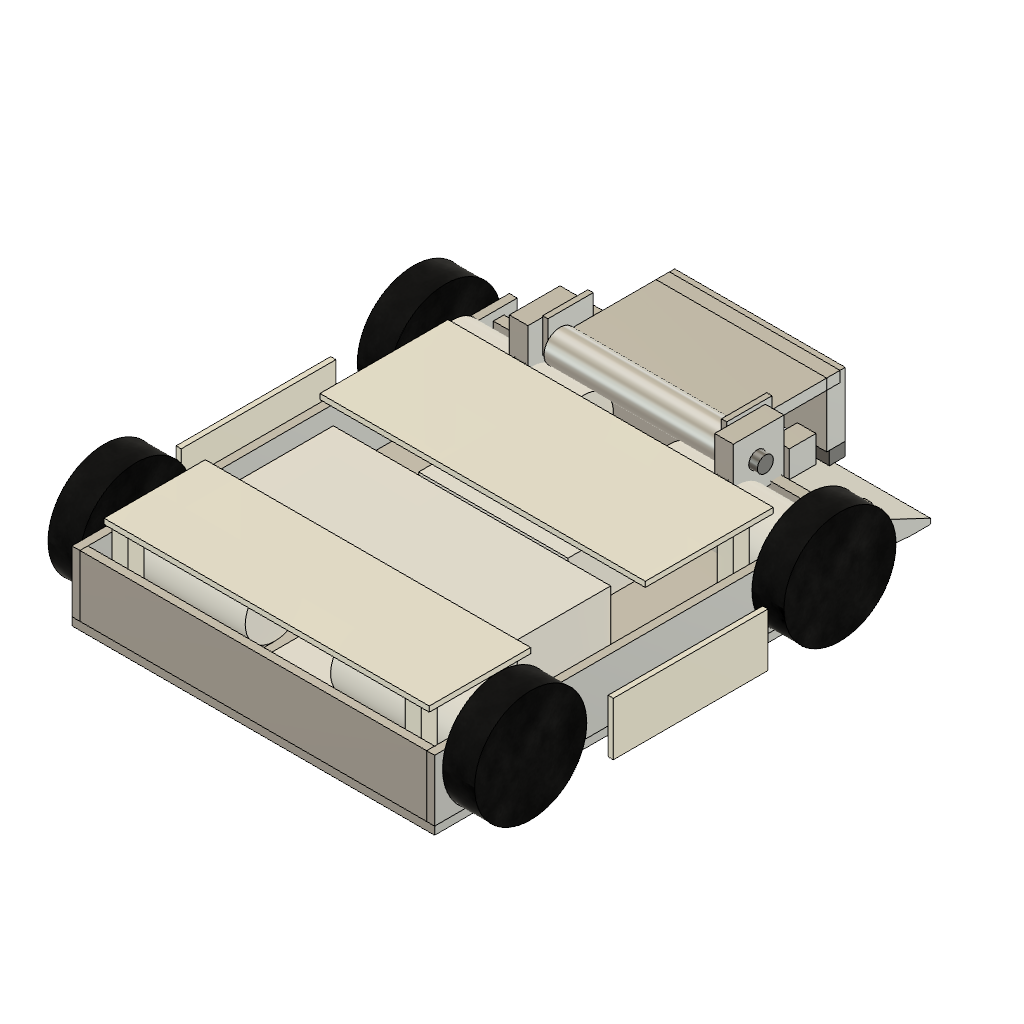
ROBOT_V3_Competition (Autodesk Fusion 360 design; units mm, degrees)
part number: 2026-09-24-19-02-37-994
part number: 2026-09-24-19-02-38-346
part number: 2026-09-24-19-02-38-350
part number: 2026-09-24-19-02-38-362
part number: 2026-09-24-19-02-38-371
part number: 2026-09-24-19-02-38-381
part number: 2026-09-24-19-02-38-392
part number: 2026-09-24-19-02-38-402
part number: 2026-09-24-19-02-38-411
part number: 2026-09-24-19-02-38-422
part number: 2026-09-24-19-02-38-425
part number: 2026-09-24-19-02-38-436
part number: 2026-09-24-19-02-38-447
part number: 2026-09-24-19-02-38-458
part number: 2026-09-24-19-02-38-470
part number: 2026-09-24-19-02-38-483
part number: 2026-09-24-19-02-38-496
part number: 2026-09-24-19-02-38-510
part number: 2026-09-24-19-02-38-525
part number: 2026-09-24-19-02-38-539
part number: 2026-09-24-19-02-38-554
part number: 2026-09-24-19-02-38-570
part number: 2026-09-24-19-02-38-586
part number: 2026-09-24-19-02-38-605
part number: 2026-09-24-19-02-38-624
part number: 2026-09-24-19-02-38-629
part number: 2026-09-24-19-02-38-655
part number: 2026-09-24-19-02-38-675
part number: 2026-09-24-19-02-38-696
part number: 2026-09-24-19-02-38-702
part number: 2026-09-24-19-02-38-753
part number: 2026-09-24-19-02-38-777
part number: 2026-09-24-19-02-38-800
part number: 2026-09-24-19-02-38-823
part number: 2026-09-24-19-02-38-847
part number: 2026-09-24-19-02-38-872
part number: 2026-09-24-19-02-38-933
part number: 2026-09-24-19-02-38-978
part number: 2026-09-24-19-02-39-006
part number: 2026-09-24-19-02-39-054
part number: 2026-09-24-19-02-39-085
part number: 2026-09-24-19-02-39-114
part number: 2026-09-24-19-02-39-145
part number: 2026-09-24-19-02-39-197
part number: 2026-09-24-19-02-39-235
part number: 2026-09-24-19-02-39-288
part number: 2026-09-24-19-02-39-435
part number: 2026-09-24-19-02-39-444
part number: 2026-09-24-19-02-39-476
part number: 2026-09-24-19-02-39-510
part number: 2026-09-24-19-02-39-543
part number: 2026-09-24-19-02-39-578
part number: 2026-09-24-19-02-39-612
part number: 2026-09-24-19-02-39-622
part number: 2026-09-24-19-02-39-658
part number: 2026-09-24-19-02-39-694
part number: 2026-09-24-19-02-39-731
part number: 2026-09-24-19-02-39-768
part number: 2026-09-24-19-02-39-806
Autodesk Fusion 360 part; units mm, degrees
sketch "Base_6061_3mm_Footprint" plane through (0, 0, 0) normal (0, 1, 0) x (1, 0, 0) in component "Base_6061_3mm"
  line L0 (-68, -82) -> (68, -82)
  line L1 (68, -82) -> (68, 82)
  line L2 (68, 82) -> (-68, 82)
  line L3 (-68, 82) -> (-68, -82)
extrude "Extrude1" add sketch "Base_6061_3mm_Footprint" along normal blind 3 from surface at 3 makes body 1 in component "Base_6061_3mm"
sketch "Side_Rail_L_6061_Footprint" plane through (0, 0, 0) normal (0, 1, 0) x (1, 0, 0) in component "Side_Rail_L_6061"
  line L0 (-68, -82) -> (-65, -82)
  line L1 (-65, -82) -> (-65, 82)
  line L2 (-65, 82) -> (-68, 82)
  line L3 (-68, 82) -> (-68, -82)
extrude "Extrude1'" add sketch "Side_Rail_L_6061_Footprint" along normal blind 23 from surface at 6 separate body makes body 2 in component "Side_Rail_L_6061"
sketch "Side_Rail_R_6061_Footprint" plane through (0, 0, 0) normal (0, 1, 0) x (1, 0, 0) in component "Side_Rail_R_6061"
  line L0 (65, -82) -> (68, -82)
  line L1 (68, -82) -> (68, 82)
  line L2 (68, 82) -> (65, 82)
  line L3 (65, 82) -> (65, -82)
extrude "Extrude1''" add sketch "Side_Rail_R_6061_Footprint" along normal blind 23 from surface at 6 separate body makes body 3 in component "Side_Rail_R_6061"
sketch "Rear_Cross_Member_6061_Footprint" plane through (0, 0, 0) normal (0, 1, 0) x (1, 0, 0) in component "Rear_Cross_Member_6061"
  line L0 (-65, -82) -> (65, -82)
  line L1 (65, -82) -> (65, -79)
  line L2 (65, -79) -> (-65, -79)
  line L3 (-65, -79) -> (-65, -82)
extrude "Extrude1'''" add sketch "Rear_Cross_Member_6061_Footprint" along normal blind 23 from surface at 6 separate body makes body 4 in component "Rear_Cross_Member_6061"
sketch "Front_Impact_Bulkhead_6061_Footprint" plane through (0, 0, 0) normal (0, 1, 0) x (1, 0, 0) in component "Front_Impact_Bulkhead_6061"
  line L0 (-62, 70) -> (62, 70)
  line L1 (62, 70) -> (62, 74)
  line L2 (62, 74) -> (-62, 74)
  line L3 (-62, 74) -> (-62, 70)
extrude "Extrude1''''" add sketch "Front_Impact_Bulkhead_6061_Footprint" along normal blind 23 from surface at 6 separate body makes body 5 in component "Front_Impact_Bulkhead_6061"
sketch "Front_Shear_Key_L_Footprint" plane through (0, 0, 0) normal (0, 1, 0) x (1, 0, 0) in component "Front_Shear_Key_L"
  line L0 (-60, 62) -> (-48, 62)
  line L1 (-48, 62) -> (-48, 70)
  line L2 (-48, 70) -> (-60, 70)
  line L3 (-60, 70) -> (-60, 62)
extrude "Extrude1'''''" add sketch "Front_Shear_Key_L_Footprint" along normal blind 18 from surface at 6 separate body makes body 6 in component "Front_Shear_Key_L"
sketch "Front_Shear_Key_R_Footprint" plane through (0, 0, 0) normal (0, 1, 0) x (1, 0, 0) in component "Front_Shear_Key_R"
  line L0 (48, 62) -> (60, 62)
  line L1 (60, 62) -> (60, 70)
  line L2 (60, 70) -> (48, 70)
  line L3 (48, 70) -> (48, 62)
extrude "Extrude1''''''" add sketch "Front_Shear_Key_R_Footprint" along normal blind 18 from surface at 6 separate body makes body 7 in component "Front_Shear_Key_R"
sketch "BBB_22mm_Gearmotor_ENVELOPE_L_Rear_Section" plane through (0, 0, 0) normal (1, 0, 0) x (0, 0, -1) in component "BBB_22mm_Gearmotor_ENVELOPE_L_Rear"
  circle A0 centre (-58, 23) radius 11
extrude "Extrude1'''''''" add sketch "BBB_22mm_Gearmotor_ENVELOPE_L_Rear_Section" along normal blind 49 from surface at -65 separate body makes body 8 in component "BBB_22mm_Gearmotor_ENVELOPE_L_Rear"
sketch "Wheel_42mm_ENVELOPE_L_Rear_Section" plane through (0, 0, 0) normal (1, 0, 0) x (0, 0, -1) in component "Wheel_42mm_ENVELOPE_L_Rear"
  circle A0 centre (-58, 23) radius 21
extrude "Extrude1''''''''" add sketch "Wheel_42mm_ENVELOPE_L_Rear_Section" along normal blind 12 from surface at -80 separate body makes body 9 in component "Wheel_42mm_ENVELOPE_L_Rear"
sketch "Axle_4mm_ENVELOPE_L_Rear_Section" plane through (0, 0, 0) normal (1, 0, 0) x (0, 0, -1) in component "Axle_4mm_ENVELOPE_L_Rear"
  circle A0 centre (-58, 23) radius 2
extrude "Extrude1'''''''''" add sketch "Axle_4mm_ENVELOPE_L_Rear_Section" along normal blind 9 from surface at -71 separate body makes body 10 in component "Axle_4mm_ENVELOPE_L_Rear"
sketch "BBB_22mm_Gearmotor_ENVELOPE_L_Front_Section" plane through (0, 0, 0) normal (1, 0, 0) x (0, 0, -1) in component "BBB_22mm_Gearmotor_ENVELOPE_L_Front"
  circle A0 centre (58, 23) radius 11
extrude "Extrude1''''''''''" add sketch "BBB_22mm_Gearmotor_ENVELOPE_L_Front_Section" along normal blind 49 from surface at -65 separate body makes body 11 in component "BBB_22mm_Gearmotor_ENVELOPE_L_Front"
sketch "Wheel_42mm_ENVELOPE_L_Front_Section" plane through (0, 0, 0) normal (1, 0, 0) x (0, 0, -1) in component "Wheel_42mm_ENVELOPE_L_Front"
  circle A0 centre (58, 23) radius 21
extrude "Extrude1'''''''''''" add sketch "Wheel_42mm_ENVELOPE_L_Front_Section" along normal blind 12 from surface at -80 separate body makes body 12 in component "Wheel_42mm_ENVELOPE_L_Front"
sketch "Axle_4mm_ENVELOPE_L_Front_Section" plane through (0, 0, 0) normal (1, 0, 0) x (0, 0, -1) in component "Axle_4mm_ENVELOPE_L_Front"
  circle A0 centre (58, 23) radius 2
extrude "Extrude1''''''''''''" add sketch "Axle_4mm_ENVELOPE_L_Front_Section" along normal blind 9 from surface at -71 separate body makes body 13 in component "Axle_4mm_ENVELOPE_L_Front"
sketch "BBB_22mm_Gearmotor_ENVELOPE_R_Rear_Section" plane through (0, 0, 0) normal (1, 0, 0) x (0, 0, -1) in component "BBB_22mm_Gearmotor_ENVELOPE_R_Rear"
  circle A0 centre (-58, 23) radius 11
extrude "Extrude1'''''''''''''" add sketch "BBB_22mm_Gearmotor_ENVELOPE_R_Rear_Section" along normal blind 49 from surface at 16 separate body makes body 14 in component "BBB_22mm_Gearmotor_ENVELOPE_R_Rear"
sketch "Wheel_42mm_ENVELOPE_R_Rear_Section" plane through (0, 0, 0) normal (1, 0, 0) x (0, 0, -1) in component "Wheel_42mm_ENVELOPE_R_Rear"
  circle A0 centre (-58, 23) radius 21
extrude "Extrude1''''''''''''''" add sketch "Wheel_42mm_ENVELOPE_R_Rear_Section" along normal blind 12 from surface at 68 separate body makes body 15 in component "Wheel_42mm_ENVELOPE_R_Rear"
sketch "Axle_4mm_ENVELOPE_R_Rear_Section" plane through (0, 0, 0) normal (1, 0, 0) x (0, 0, -1) in component "Axle_4mm_ENVELOPE_R_Rear"
  circle A0 centre (-58, 23) radius 2
extrude "Extrude1'''''''''''''''" add sketch "Axle_4mm_ENVELOPE_R_Rear_Section" along normal blind 9 from surface at 62 separate body makes body 16 in component "Axle_4mm_ENVELOPE_R_Rear"
sketch "BBB_22mm_Gearmotor_ENVELOPE_R_Front_Section" plane through (0, 0, 0) normal (1, 0, 0) x (0, 0, -1) in component "BBB_22mm_Gearmotor_ENVELOPE_R_Front"
  circle A0 centre (58, 23) radius 11
extrude "Extrude1''''''''''''''''" add sketch "BBB_22mm_Gearmotor_ENVELOPE_R_Front_Section" along normal blind 49 from surface at 16 separate body makes body 17 in component "BBB_22mm_Gearmotor_ENVELOPE_R_Front"
sketch "Wheel_42mm_ENVELOPE_R_Front_Section" plane through (0, 0, 0) normal (1, 0, 0) x (0, 0, -1) in component "Wheel_42mm_ENVELOPE_R_Front"
  circle A0 centre (58, 23) radius 21
extrude "Extrude1'''''''''''''''''" add sketch "Wheel_42mm_ENVELOPE_R_Front_Section" along normal blind 12 from surface at 68 separate body makes body 18 in component "Wheel_42mm_ENVELOPE_R_Front"
sketch "Axle_4mm_ENVELOPE_R_Front_Section" plane through (0, 0, 0) normal (1, 0, 0) x (0, 0, -1) in component "Axle_4mm_ENVELOPE_R_Front"
  circle A0 centre (58, 23) radius 2
extrude "Extrude1''''''''''''''''''" add sketch "Axle_4mm_ENVELOPE_R_Front_Section" along normal blind 9 from surface at 62 separate body makes body 19 in component "Axle_4mm_ENVELOPE_R_Front"
sketch "Replaceable_Side_Guard_L_Footprint" plane through (0, 0, 0) normal (0, 1, 0) x (1, 0, 0) in component "Replaceable_Side_Guard_L"
  line L0 (-82, -29) -> (-80, -29)
  line L1 (-80, -29) -> (-80, 29)
  line L2 (-80, 29) -> (-82, 29)
  line L3 (-82, 29) -> (-82, -29)
extrude "Extrude1'''''''''''''''''''" add sketch "Replaceable_Side_Guard_L_Footprint" along normal blind 20 from surface at 8 separate body makes body 20 in component "Replaceable_Side_Guard_L"
sketch "Replaceable_Side_Guard_R_Footprint" plane through (0, 0, 0) normal (0, 1, 0) x (1, 0, 0) in component "Replaceable_Side_Guard_R"
  line L0 (80, -29) -> (82, -29)
  line L1 (82, -29) -> (82, 29)
  line L2 (82, 29) -> (80, 29)
  line L3 (80, 29) -> (80, -29)
extrude "Extrude1''''''''''''''''''''" add sketch "Replaceable_Side_Guard_R_Footprint" along normal blind 20 from surface at 8 separate body makes body 21 in component "Replaceable_Side_Guard_R"
sketch "Plow_Ramp_Profile" plane through (0, 0, 0) normal (1, 0, 0) x (0, 0, -1) in component "Bolt_On_Full_Width_Plow_6061"
  line L0 (74, 6) -> (74, 23)
  line L1 (74, 23) -> (112, 5)
  line L2 (112, 5) -> (112, 3)
  line L3 (112, 3) -> (104, 3)
  line L4 (104, 3) -> (74, 6)
extrude "Extrude1'''''''''''''''''''''" add sketch "Plow_Ramp_Profile" along normal blind 120 from surface at -60 separate body makes body 22 in component "Bolt_On_Full_Width_Plow_6061"
sketch "Plow_Bolt_Land_L_Footprint" plane through (0, 0, 0) normal (0, 1, 0) x (1, 0, 0) in component "Plow_Bolt_Land_L"
  line L0 (-54, 65) -> (-44, 65)
  line L1 (-44, 65) -> (-44, 74)
  line L2 (-44, 74) -> (-54, 74)
  line L3 (-54, 74) -> (-54, 65)
extrude "Extrude1''''''''''''''''''''''" add sketch "Plow_Bolt_Land_L_Footprint" along normal blind 16 from surface at 6 separate body makes body 23 in component "Plow_Bolt_Land_L"
sketch "Plow_Bolt_Land_R_Footprint" plane through (0, 0, 0) normal (0, 1, 0) x (1, 0, 0) in component "Plow_Bolt_Land_R"
  line L0 (44, 65) -> (54, 65)
  line L1 (54, 65) -> (54, 74)
  line L2 (54, 74) -> (44, 74)
  line L3 (44, 74) -> (44, 65)
extrude "Extrude1'''''''''''''''''''''''" add sketch "Plow_Bolt_Land_R_Footprint" along normal blind 16 from surface at 6 separate body makes body 24 in component "Plow_Bolt_Land_R"
sketch "Clamp_Jaw_Plate_6061_Footprint" plane through (0, 0, 0) normal (0, 1, 0) x (1, 0, 0) in component "Clamp_Jaw_Plate_6061"
  line L0 (-32, 65) -> (32, 65)
  line L1 (32, 65) -> (32, 106)
  line L2 (32, 106) -> (-32, 106)
  line L3 (-32, 106) -> (-32, 65)
extrude "Extrude1''''''''''''''''''''''''" add sketch "Clamp_Jaw_Plate_6061_Footprint" along normal blind 4 from surface at 38 separate body makes body 25 in component "Clamp_Jaw_Plate_6061"
sketch "Hinge_Boss_Section" plane through (0, 0, 0) normal (1, 0, 0) x (0, 0, -1) in component "Clamp_Jaw_Plate_6061"
  circle A0 centre (65, 38.5) radius 6
extrude "Extrude2" add sketch "Hinge_Boss_Section" along normal blind 64 from surface at -32 bodies 25 in component "Clamp_Jaw_Plate_6061"
sketch "Hinge_Bore_6p4mm" plane through (0, 0, 0) normal (1, 0, 0) x (0, 0, -1) in component "Clamp_Jaw_Plate_6061"
  circle A0 centre (65, 38.5) radius 3.2
extrude "Extrude3" cut sketch "Hinge_Bore_6p4mm" along normal mid plane 200 bodies 25 in component "Clamp_Jaw_Plate_6061"
sketch "Clamp_Downturned_Tip_6061_Footprint" plane through (0, 0, 0) normal (0, 1, 0) x (1, 0, 0) in component "Clamp_Downturned_Tip_6061"
  line L0 (-32, 101) -> (32, 101)
  line L1 (32, 101) -> (32, 108)
  line L2 (32, 108) -> (-32, 108)
  line L3 (-32, 108) -> (-32, 101)
extrude "Extrude1'''''''''''''''''''''''''" add sketch "Clamp_Downturned_Tip_6061_Footprint" along normal blind 24 from surface at 18 separate body makes body 26 in component "Clamp_Downturned_Tip_6061"
sketch "Replaceable_Clamp_Tooth_1_Steel_Footprint" plane through (0, 0, 0) normal (0, 1, 0) x (1, 0, 0) in component "Replaceable_Clamp_Tooth_1_Steel"
  line L0 (-28, 106) -> (-20, 106)
  line L1 (-20, 106) -> (-20, 112)
  line L2 (-20, 112) -> (-28, 112)
  line L3 (-28, 112) -> (-28, 106)
extrude "Extrude1''''''''''''''''''''''''''" add sketch "Replaceable_Clamp_Tooth_1_Steel_Footprint" along normal blind 11 from surface at 9 separate body makes body 27 in component "Replaceable_Clamp_Tooth_1_Steel"
sketch "Replaceable_Clamp_Tooth_2_Steel_Footprint" plane through (0, 0, 0) normal (0, 1, 0) x (1, 0, 0) in component "Replaceable_Clamp_Tooth_2_Steel"
  line L0 (-4, 106) -> (4, 106)
  line L1 (4, 106) -> (4, 112)
  line L2 (4, 112) -> (-4, 112)
  line L3 (-4, 112) -> (-4, 106)
extrude "Extrude1'''''''''''''''''''''''''''" add sketch "Replaceable_Clamp_Tooth_2_Steel_Footprint" along normal blind 11 from surface at 9 separate body makes body 28 in component "Replaceable_Clamp_Tooth_2_Steel"
sketch "Replaceable_Clamp_Tooth_3_Steel_Footprint" plane through (0, 0, 0) normal (0, 1, 0) x (1, 0, 0) in component "Replaceable_Clamp_Tooth_3_Steel"
  line L0 (20, 106) -> (28, 106)
  line L1 (28, 106) -> (28, 112)
  line L2 (28, 112) -> (20, 112)
  line L3 (20, 112) -> (20, 106)
extrude "Extrude1''''''''''''''''''''''''''''" add sketch "Replaceable_Clamp_Tooth_3_Steel_Footprint" along normal blind 11 from surface at 9 separate body makes body 29 in component "Replaceable_Clamp_Tooth_3_Steel"
sketch "Clamp_Torque_Arm_L_Footprint" plane through (0, 0, 0) normal (0, 1, 0) x (1, 0, 0) in component "Clamp_Torque_Arm_L"
  line L0 (-34.5, 61) -> (-32.5, 61)
  line L1 (-32.5, 61) -> (-32.5, 78)
  line L2 (-32.5, 78) -> (-34.5, 78)
  line L3 (-34.5, 78) -> (-34.5, 61)
extrude "Extrude1'''''''''''''''''''''''''''''" add sketch "Clamp_Torque_Arm_L_Footprint" along normal blind 13 from surface at 36 separate body makes body 30 in component "Clamp_Torque_Arm_L"
sketch "Clamp_Torque_Arm_R_Footprint" plane through (0, 0, 0) normal (0, 1, 0) x (1, 0, 0) in component "Clamp_Torque_Arm_R"
  line L0 (32.5, 61) -> (34.5, 61)
  line L1 (34.5, 61) -> (34.5, 78)
  line L2 (34.5, 78) -> (32.5, 78)
  line L3 (32.5, 78) -> (32.5, 61)
extrude "Extrude1''''''''''''''''''''''''''''''" add sketch "Clamp_Torque_Arm_R_Footprint" along normal blind 13 from surface at 36 separate body makes body 31 in component "Clamp_Torque_Arm_R"
sketch "Torque_Arm_Pin_Bore_L" plane through (0, 0, 0) normal (1, 0, 0) x (0, 0, -1) in component "Clamp_Torque_Arm_L"
  circle A0 centre (65, 38.5) radius 3.2
extrude "Extrude2'" cut sketch "Torque_Arm_Pin_Bore_L" along normal mid plane 200 bodies 30 in component "Clamp_Torque_Arm_L"
sketch "Torque_Arm_Pin_Bore_R" plane through (0, 0, 0) normal (1, 0, 0) x (0, 0, -1) in component "Clamp_Torque_Arm_R"
  circle A0 centre (65, 38.5) radius 3.2
extrude "Extrude2''" cut sketch "Torque_Arm_Pin_Bore_R" along normal mid plane 200 bodies 31 in component "Clamp_Torque_Arm_R"
sketch "Hinge_Cheek_L_Footprint" plane through (0, 0, 0) normal (0, 1, 0) x (1, 0, 0) in component "Hinge_Cheek_L"
  line L0 (-42, 56) -> (-35, 56)
  line L1 (-35, 56) -> (-35, 75)
  line L2 (-35, 75) -> (-42, 75)
  line L3 (-42, 75) -> (-42, 56)
extrude "Extrude1'''''''''''''''''''''''''''''''" add sketch "Hinge_Cheek_L_Footprint" along normal blind 20 from surface at 28 separate body makes body 32 in component "Hinge_Cheek_L"
sketch "Pin_Bore_6p4mm" plane through (0, 0, 0) normal (1, 0, 0) x (0, 0, -1) in component "Hinge_Cheek_L"
  circle A0 centre (65, 38.5) radius 3.2
extrude "Extrude2'''" cut sketch "Pin_Bore_6p4mm" along normal mid plane 200 bodies 32 in component "Hinge_Cheek_L"
sketch "Downward_Hard_Stop_L_Footprint" plane through (0, 0, 0) normal (0, 1, 0) x (1, 0, 0) in component "Downward_Hard_Stop_L"
  line L0 (-42, 77) -> (-35, 77)
  line L1 (-35, 77) -> (-35, 87)
  line L2 (-35, 87) -> (-42, 87)
  line L3 (-42, 87) -> (-42, 77)
extrude "Extrude1''''''''''''''''''''''''''''''''" add sketch "Downward_Hard_Stop_L_Footprint" along normal blind 10 from surface at 26 separate body makes body 33 in component "Downward_Hard_Stop_L"
sketch "Hinge_Cheek_R_Footprint" plane through (0, 0, 0) normal (0, 1, 0) x (1, 0, 0) in component "Hinge_Cheek_R"
  line L0 (35, 56) -> (42, 56)
  line L1 (42, 56) -> (42, 75)
  line L2 (42, 75) -> (35, 75)
  line L3 (35, 75) -> (35, 56)
extrude "Extrude1'''''''''''''''''''''''''''''''''" add sketch "Hinge_Cheek_R_Footprint" along normal blind 20 from surface at 28 separate body makes body 34 in component "Hinge_Cheek_R"
sketch "Pin_Bore_6p4mm (2)" plane through (0, 0, 0) normal (1, 0, 0) x (0, 0, -1) in component "Hinge_Cheek_R"
  circle A0 centre (65, 38.5) radius 3.2
extrude "Extrude2''''" cut sketch "Pin_Bore_6p4mm (2)" along normal mid plane 200 bodies 34 in component "Hinge_Cheek_R"
sketch "Downward_Hard_Stop_R_Footprint" plane through (0, 0, 0) normal (0, 1, 0) x (1, 0, 0) in component "Downward_Hard_Stop_R"
  line L0 (35, 77) -> (42, 77)
  line L1 (42, 77) -> (42, 87)
  line L2 (42, 87) -> (35, 87)
  line L3 (35, 87) -> (35, 77)
extrude "Extrude1''''''''''''''''''''''''''''''''''" add sketch "Downward_Hard_Stop_R_Footprint" along normal blind 10 from surface at 26 separate body makes body 35 in component "Downward_Hard_Stop_R"
sketch "Hinge_Pin_6mm_ENVELOPE_Section" plane through (0, 0, 0) normal (1, 0, 0) x (0, 0, -1) in component "Hinge_Pin_6mm_ENVELOPE"
  circle A0 centre (65, 38.5) radius 3
extrude "Extrude1'''''''''''''''''''''''''''''''''''" add sketch "Hinge_Pin_6mm_ENVELOPE_Section" along normal blind 90 from surface at -45 separate body makes body 36 in component "Hinge_Pin_6mm_ENVELOPE"
sketch "Repeat_40kg_Servo_ENVELOPE_Footprint" plane through (0, 0, 0) normal (0, 1, 0) x (1, 0, 0) in component "Repeat_40kg_Servo_ENVELOPE"
  line L0 (-28, 8) -> (28, 8)
  line L1 (28, 8) -> (28, 53)
  line L2 (28, 53) -> (-28, 53)
  line L3 (-28, 53) -> (-28, 8)
extrude "Extrude1''''''''''''''''''''''''''''''''''''" add sketch "Repeat_40kg_Servo_ENVELOPE_Footprint" along normal blind 20 from surface at 8 separate body makes body 37 in component "Repeat_40kg_Servo_ENVELOPE"
sketch "Servo_Output_Horn_6061_Section" plane through (0, 0, 0) normal (1, 0, 0) x (0, 0, -1) in component "Servo_Output_Horn_6061"
  circle A0 centre (51, 24) radius 6
extrude "Extrude1'''''''''''''''''''''''''''''''''''''" add sketch "Servo_Output_Horn_6061_Section" along normal blind 68 from surface at -34 separate body makes body 38 in component "Servo_Output_Horn_6061"
sketch "Servo_Output_Bore_3mm" plane through (0, 0, 0) normal (1, 0, 0) x (0, 0, -1) in component "Servo_Output_Horn_6061"
  circle A0 centre (51, 24) radius 1.5
extrude "Extrude2'''''" cut sketch "Servo_Output_Bore_3mm" along normal mid plane 200 bodies 38 in component "Servo_Output_Horn_6061"
sketch "Sketch1" plane through (0, 0, 0) normal (1, 0, 0) x (0, 0, -1) in component "Clamp_Linkage_L"
  line L0 (49.427, 29.9431) -> (70.427, 46.9431)
  line L1 (70.427, 46.9431) -> (73.573, 43.0569)
  line L2 (73.573, 43.0569) -> (52.573, 26.0569)
  line L3 (52.573, 26.0569) -> (49.427, 29.9431)
extrude "Extrude1''''''''''''''''''''''''''''''''''''''" add sketch "Sketch1" along normal blind 4 from surface at -40 separate body makes body 39 in component "Clamp_Linkage_L"
sketch "Sketch1 (2)" plane through (0, 0, 0) normal (1, 0, 0) x (0, 0, -1) in component "Clamp_Linkage_R"
  line L0 (49.427, 29.9431) -> (70.427, 46.9431)
  line L1 (70.427, 46.9431) -> (73.573, 43.0569)
  line L2 (73.573, 43.0569) -> (52.573, 26.0569)
  line L3 (52.573, 26.0569) -> (49.427, 29.9431)
extrude "Extrude1'''''''''''''''''''''''''''''''''''''''" add sketch "Sketch1 (2)" along normal blind 4 from surface at 36 separate body makes body 40 in component "Clamp_Linkage_R"
sketch "Servo_Linkage_Sweep_ENVELOPE_Footprint" plane through (0, 0, 0) normal (0, 1, 0) x (1, 0, 0) in component "Servo_Linkage_Sweep_ENVELOPE"
  line L0 (-9, 48) -> (9, 48)
  line L1 (9, 48) -> (9, 75)
  line L2 (9, 75) -> (-9, 75)
  line L3 (-9, 75) -> (-9, 48)
extrude "Extrude1''''''''''''''''''''''''''''''''''''''''" add sketch "Servo_Linkage_Sweep_ENVELOPE_Footprint" along normal blind 22 from surface at 28 separate body makes body 41 in component "Servo_Linkage_Sweep_ENVELOPE"
sketch "3S_Battery_104x35x27_ENVELOPE_Footprint" plane through (0, 0, 0) normal (0, 1, 0) x (1, 0, 0) in component "3S_Battery_104x35x27_ENVELOPE"
  line L0 (-52, -35) -> (52, -35)
  line L1 (52, -35) -> (52, 0)
  line L2 (52, 0) -> (-52, 0)
  line L3 (-52, 0) -> (-52, -35)
extrude "Extrude1'''''''''''''''''''''''''''''''''''''''''" add sketch "3S_Battery_104x35x27_ENVELOPE_Footprint" along normal blind 27 from surface at 8 separate body makes body 42 in component "3S_Battery_104x35x27_ENVELOPE"
sketch "Dual_ESC_ENVELOPE_Footprint" plane through (0, 0, 0) normal (0, 1, 0) x (1, 0, 0) in component "Dual_ESC_ENVELOPE"
  line L0 (-12, -72) -> (12, -72)
  line L1 (12, -72) -> (12, -52)
  line L2 (12, -52) -> (-12, -52)
  line L3 (-12, -52) -> (-12, -72)
extrude "Extrude1''''''''''''''''''''''''''''''''''''''''''" add sketch "Dual_ESC_ENVELOPE_Footprint" along normal blind 5 from surface at 8 separate body makes body 43 in component "Dual_ESC_ENVELOPE"
sketch "Receiver_ENVELOPE_Footprint" plane through (0, 0, 0) normal (0, 1, 0) x (1, 0, 0) in component "Receiver_ENVELOPE"
  line L0 (-48, -72) -> (-20, -72)
  line L1 (-20, -72) -> (-20, -54)
  line L2 (-20, -54) -> (-48, -54)
  line L3 (-48, -54) -> (-48, -72)
extrude "Extrude1'''''''''''''''''''''''''''''''''''''''''''" add sketch "Receiver_ENVELOPE_Footprint" along normal blind 6 from surface at 8 separate body makes body 44 in component "Receiver_ENVELOPE"
sketch "UBEC_ENVELOPE_Footprint" plane through (0, 0, 0) normal (0, 1, 0) x (1, 0, 0) in component "UBEC_ENVELOPE"
  line L0 (20, -72) -> (48, -72)
  line L1 (48, -72) -> (48, -54)
  line L2 (48, -54) -> (20, -54)
  line L3 (20, -54) -> (20, -72)
extrude "Extrude1''''''''''''''''''''''''''''''''''''''''''''" add sketch "UBEC_ENVELOPE_Footprint" along normal blind 7 from surface at 8 separate body makes body 45 in component "UBEC_ENVELOPE"
sketch "Power_Switch_ENVELOPE_Footprint" plane through (0, 0, 0) normal (0, 1, 0) x (1, 0, 0) in component "Power_Switch_ENVELOPE"
  line L0 (38, -65) -> (56, -65)
  line L1 (56, -65) -> (56, -45)
  line L2 (56, -45) -> (38, -45)
  line L3 (38, -45) -> (38, -65)
extrude "Extrude1'''''''''''''''''''''''''''''''''''''''''''''" add sketch "Power_Switch_ENVELOPE_Footprint" along normal blind 16 from surface at 9 separate body makes body 46 in component "Power_Switch_ENVELOPE"
sketch "Cover_Standoff_L_Rear_Footprint" plane through (0, 0, 0) normal (0, 1, 0) x (1, 0, 0) in component "Cover_Standoff_L_Rear"
  line L0 (-58, -77) -> (-52, -77)
  line L1 (-52, -77) -> (-52, -71)
  line L2 (-52, -71) -> (-58, -71)
  line L3 (-58, -71) -> (-58, -77)
extrude "Extrude1''''''''''''''''''''''''''''''''''''''''''''''" add sketch "Cover_Standoff_L_Rear_Footprint" along normal blind 31 from surface at 6 separate body makes body 47 in component "Cover_Standoff_L_Rear"
sketch "Cover_Standoff_L_Front_Footprint" plane through (0, 0, 0) normal (0, 1, 0) x (1, 0, 0) in component "Cover_Standoff_L_Front"
  line L0 (-58, 40) -> (-52, 40)
  line L1 (-52, 40) -> (-52, 46)
  line L2 (-52, 46) -> (-58, 46)
  line L3 (-58, 46) -> (-58, 40)
extrude "Extrude1'''''''''''''''''''''''''''''''''''''''''''''''" add sketch "Cover_Standoff_L_Front_Footprint" along normal blind 31 from surface at 6 separate body makes body 48 in component "Cover_Standoff_L_Front"
sketch "Cover_Standoff_R_Rear_Footprint" plane through (0, 0, 0) normal (0, 1, 0) x (1, 0, 0) in component "Cover_Standoff_R_Rear"
  line L0 (52, -77) -> (58, -77)
  line L1 (58, -77) -> (58, -71)
  line L2 (58, -71) -> (52, -71)
  line L3 (52, -71) -> (52, -77)
extrude "Extrude1''''''''''''''''''''''''''''''''''''''''''''''''" add sketch "Cover_Standoff_R_Rear_Footprint" along normal blind 31 from surface at 6 separate body makes body 49 in component "Cover_Standoff_R_Rear"
sketch "Cover_Standoff_R_Front_Footprint" plane through (0, 0, 0) normal (0, 1, 0) x (1, 0, 0) in component "Cover_Standoff_R_Front"
  line L0 (52, 40) -> (58, 40)
  line L1 (58, 40) -> (58, 46)
  line L2 (58, 46) -> (52, 46)
  line L3 (52, 46) -> (52, 40)
extrude "Extrude1'''''''''''''''''''''''''''''''''''''''''''''''''" add sketch "Cover_Standoff_R_Front_Footprint" along normal blind 31 from surface at 6 separate body makes body 50 in component "Cover_Standoff_R_Front"
sketch "Rear_Service_Lid_2mm_Footprint" plane through (0, 0, 0) normal (0, 1, 0) x (1, 0, 0) in component "Rear_Service_Lid_2mm"
  line L0 (-61, -77) -> (61, -77)
  line L1 (61, -77) -> (61, -39)
  line L2 (61, -39) -> (-61, -39)
  line L3 (-61, -39) -> (-61, -77)
extrude "Extrude1''''''''''''''''''''''''''''''''''''''''''''''''''" add sketch "Rear_Service_Lid_2mm_Footprint" along normal blind 2 from surface at 37 separate body makes body 51 in component "Rear_Service_Lid_2mm"
sketch "Center_Service_Lid_2mm_Footprint" plane through (0, 0, 0) normal (0, 1, 0) x (1, 0, 0) in component "Center_Service_Lid_2mm"
  line L0 (-61, 4) -> (61, 4)
  line L1 (61, 4) -> (61, 52)
  line L2 (61, 52) -> (-61, 52)
  line L3 (-61, 52) -> (-61, 4)
extrude "Extrude1'''''''''''''''''''''''''''''''''''''''''''''''''''" add sketch "Center_Service_Lid_2mm_Footprint" along normal blind 2 from surface at 37 separate body makes body 52 in component "Center_Service_Lid_2mm"
component "01_Low_Tub_Chassis" placed x (1, 0, 0) y (0, 1, 0) z (0, 0, 1) at (0, 0, 0)
component "02_Four_Wheel_Drive" placed x (1, 0, 0) y (0, 1, 0) z (0, 0, 1) at (0, 0, 0)
component "03_Front_Impact_Module" placed x (1, 0, 0) y (0, 1, 0) z (0, 0, 1) at (0, 0, 0)
component "04_Protected_Clamp_Weapon" placed x (1, 0, 0) y (0, 1, 0) z (0, 0, 1) at (0, 0, 0)
component "05_Protected_Electronics_ENVELOPES" placed x (1, 0, 0) y (0, 1, 0) z (0, 0, 1) at (0, 0, 0)
component "06_Removable_Covers" placed x (1, 0, 0) y (0, 1, 0) z (0, 0, 1) at (0, 0, 0)
component "Base_6061_3mm" placed x (1, 0, 0) y (0, 1, 0) z (0, 0, 1) at (0, 0, 0) in component "01_Low_Tub_Chassis"
component "Side_Rail_L_6061" placed x (1, 0, 0) y (0, 1, 0) z (0, 0, 1) at (0, 0, 0) in component "01_Low_Tub_Chassis"
component "Side_Rail_R_6061" placed x (1, 0, 0) y (0, 1, 0) z (0, 0, 1) at (0, 0, 0) in component "01_Low_Tub_Chassis"
component "Rear_Cross_Member_6061" placed x (1, 0, 0) y (0, 1, 0) z (0, 0, 1) at (0, 0, 0) in component "01_Low_Tub_Chassis"
component "Front_Impact_Bulkhead_6061" placed x (1, 0, 0) y (0, 1, 0) z (0, 0, 1) at (0, 0, 0) in component "01_Low_Tub_Chassis"
component "Front_Shear_Key_L" placed x (1, 0, 0) y (0, 1, 0) z (0, 0, 1) at (0, 0, 0) in component "01_Low_Tub_Chassis"
component "Front_Shear_Key_R" placed x (1, 0, 0) y (0, 1, 0) z (0, 0, 1) at (0, 0, 0) in component "01_Low_Tub_Chassis"
component "BBB_22mm_Gearmotor_ENVELOPE_L_Rear" placed x (1, 0, 0) y (0, 1, 0) z (0, 0, 1) at (0, 0, 0) in component "02_Four_Wheel_Drive"
component "Wheel_42mm_ENVELOPE_L_Rear" placed x (1, 0, 0) y (0, 1, 0) z (0, 0, 1) at (0, 0, 0) in component "02_Four_Wheel_Drive"
component "Axle_4mm_ENVELOPE_L_Rear" placed x (1, 0, 0) y (0, 1, 0) z (0, 0, 1) at (0, 0, 0) in component "02_Four_Wheel_Drive"
component "BBB_22mm_Gearmotor_ENVELOPE_L_Front" placed x (1, 0, 0) y (0, 1, 0) z (0, 0, 1) at (0, 0, 0) in component "02_Four_Wheel_Drive"
component "Wheel_42mm_ENVELOPE_L_Front" placed x (1, 0, 0) y (0, 1, 0) z (0, 0, 1) at (0, 0, 0) in component "02_Four_Wheel_Drive"
component "Axle_4mm_ENVELOPE_L_Front" placed x (1, 0, 0) y (0, 1, 0) z (0, 0, 1) at (0, 0, 0) in component "02_Four_Wheel_Drive"
component "BBB_22mm_Gearmotor_ENVELOPE_R_Rear" placed x (1, 0, 0) y (0, 1, 0) z (0, 0, 1) at (0, 0, 0) in component "02_Four_Wheel_Drive"
component "Wheel_42mm_ENVELOPE_R_Rear" placed x (1, 0, 0) y (0, 1, 0) z (0, 0, 1) at (0, 0, 0) in component "02_Four_Wheel_Drive"
component "Axle_4mm_ENVELOPE_R_Rear" placed x (1, 0, 0) y (0, 1, 0) z (0, 0, 1) at (0, 0, 0) in component "02_Four_Wheel_Drive"
component "BBB_22mm_Gearmotor_ENVELOPE_R_Front" placed x (1, 0, 0) y (0, 1, 0) z (0, 0, 1) at (0, 0, 0) in component "02_Four_Wheel_Drive"
component "Wheel_42mm_ENVELOPE_R_Front" placed x (1, 0, 0) y (0, 1, 0) z (0, 0, 1) at (0, 0, 0) in component "02_Four_Wheel_Drive"
component "Axle_4mm_ENVELOPE_R_Front" placed x (1, 0, 0) y (0, 1, 0) z (0, 0, 1) at (0, 0, 0) in component "02_Four_Wheel_Drive"
component "Replaceable_Side_Guard_L" placed x (1, 0, 0) y (0, 1, 0) z (0, 0, 1) at (0, 0, 0) in component "02_Four_Wheel_Drive"
component "Replaceable_Side_Guard_R" placed x (1, 0, 0) y (0, 1, 0) z (0, 0, 1) at (0, 0, 0) in component "02_Four_Wheel_Drive"
component "Bolt_On_Full_Width_Plow_6061" placed x (1, 0, 0) y (0, 1, 0) z (0, 0, 1) at (0, 0, 0) in component "03_Front_Impact_Module"
component "Plow_Bolt_Land_L" placed x (1, 0, 0) y (0, 1, 0) z (0, 0, 1) at (0, 0, 0) in component "03_Front_Impact_Module"
component "Plow_Bolt_Land_R" placed x (1, 0, 0) y (0, 1, 0) z (0, 0, 1) at (0, 0, 0) in component "03_Front_Impact_Module"
component "Clamp_Jaw_Plate_6061" placed x (1, 0, 0) y (0, 1, 0) z (0, 0, 1) at (0, 0, 0) in component "04_Protected_Clamp_Weapon"
component "Clamp_Downturned_Tip_6061" placed x (1, 0, 0) y (0, 1, 0) z (0, 0, 1) at (0, 0, 0) in component "04_Protected_Clamp_Weapon"
component "Replaceable_Clamp_Tooth_1_Steel" placed x (1, 0, 0) y (0, 1, 0) z (0, 0, 1) at (0, 0, 0) in component "04_Protected_Clamp_Weapon"
component "Replaceable_Clamp_Tooth_2_Steel" placed x (1, 0, 0) y (0, 1, 0) z (0, 0, 1) at (0, 0, 0) in component "04_Protected_Clamp_Weapon"
component "Replaceable_Clamp_Tooth_3_Steel" placed x (1, 0, 0) y (0, 1, 0) z (0, 0, 1) at (0, 0, 0) in component "04_Protected_Clamp_Weapon"
component "Clamp_Torque_Arm_L" placed x (1, 0, 0) y (0, 1, 0) z (0, 0, 1) at (0, 0, 0) in component "04_Protected_Clamp_Weapon"
component "Clamp_Torque_Arm_R" placed x (1, 0, 0) y (0, 1, 0) z (0, 0, 1) at (0, 0, 0) in component "04_Protected_Clamp_Weapon"
component "Hinge_Cheek_L" placed x (1, 0, 0) y (0, 1, 0) z (0, 0, 1) at (0, 0, 0) in component "04_Protected_Clamp_Weapon"
component "Downward_Hard_Stop_L" placed x (1, 0, 0) y (0, 1, 0) z (0, 0, 1) at (0, 0, 0) in component "04_Protected_Clamp_Weapon"
component "Hinge_Cheek_R" placed x (1, 0, 0) y (0, 1, 0) z (0, 0, 1) at (0, 0, 0) in component "04_Protected_Clamp_Weapon"
component "Downward_Hard_Stop_R" placed x (1, 0, 0) y (0, 1, 0) z (0, 0, 1) at (0, 0, 0) in component "04_Protected_Clamp_Weapon"
component "Hinge_Pin_6mm_ENVELOPE" placed x (1, 0, 0) y (0, 1, 0) z (0, 0, 1) at (0, 0, 0) in component "04_Protected_Clamp_Weapon"
component "Repeat_40kg_Servo_ENVELOPE" placed x (1, 0, 0) y (0, 1, 0) z (0, 0, 1) at (0, 0, 0) in component "04_Protected_Clamp_Weapon"
component "Servo_Output_Horn_6061" placed x (1, 0, 0) y (0, 1, 0) z (0, 0, 1) at (0, 0, 0) in component "04_Protected_Clamp_Weapon"
component "Clamp_Linkage_L" placed x (1, 0, 0) y (0, 1, 0) z (0, 0, 1) at (0, 0, 0) in component "04_Protected_Clamp_Weapon"
component "Clamp_Linkage_R" placed x (1, 0, 0) y (0, 1, 0) z (0, 0, 1) at (0, 0, 0) in component "04_Protected_Clamp_Weapon"
component "Servo_Linkage_Sweep_ENVELOPE" placed x (1, 0, 0) y (0, 1, 0) z (0, 0, 1) at (0, 0, 0) in component "04_Protected_Clamp_Weapon"
component "Base_6061_3mm" placed x (1, 0, 0) y (0, 1, 0) z (0, 0, 1) at (0, 0, 0) in component "Hinge_Pin_6mm_ENVELOPE"
component "3S_Battery_104x35x27_ENVELOPE" placed x (1, 0, 0) y (0, 1, 0) z (0, 0, 1) at (0, 0, 0) in component "05_Protected_Electronics_ENVELOPES"
component "Dual_ESC_ENVELOPE" placed x (1, 0, 0) y (0, 1, 0) z (0, 0, 1) at (0, 0, 0) in component "05_Protected_Electronics_ENVELOPES"
component "Receiver_ENVELOPE" placed x (1, 0, 0) y (0, 1, 0) z (0, 0, 1) at (0, 0, 0) in component "05_Protected_Electronics_ENVELOPES"
component "UBEC_ENVELOPE" placed x (1, 0, 0) y (0, 1, 0) z (0, 0, 1) at (0, 0, 0) in component "05_Protected_Electronics_ENVELOPES"
component "Power_Switch_ENVELOPE" placed x (1, 0, 0) y (0, 1, 0) z (0, 0, 1) at (0, 0, 0) in component "05_Protected_Electronics_ENVELOPES"
component "Cover_Standoff_L_Rear" placed x (1, 0, 0) y (0, 1, 0) z (0, 0, 1) at (0, 0, 0) in component "06_Removable_Covers"
component "Cover_Standoff_L_Front" placed x (1, 0, 0) y (0, 1, 0) z (0, 0, 1) at (0, 0, 0) in component "06_Removable_Covers"
component "Cover_Standoff_R_Rear" placed x (1, 0, 0) y (0, 1, 0) z (0, 0, 1) at (0, 0, 0) in component "06_Removable_Covers"
component "Cover_Standoff_R_Front" placed x (1, 0, 0) y (0, 1, 0) z (0, 0, 1) at (0, 0, 0) in component "06_Removable_Covers"
component "Rear_Service_Lid_2mm" placed x (1, 0, 0) y (0, 1, 0) z (0, 0, 1) at (0, 0, 0) in component "06_Removable_Covers"
component "Center_Service_Lid_2mm" placed x (1, 0, 0) y (0, 1, 0) z (0, 0, 1) at (0, 0, 0) in component "06_Removable_Covers"
hidden bodies 41
named bodies: "Base_6061_3mm", "Side_Rail_L_6061", "Side_Rail_R_6061", "Rear_Cross_Member_6061", "Front_Impact_Bulkhead_6061", "Front_Shear_Key_L", "Front_Shear_Key_R", "BBB_22mm_Gearmotor_ENVELOPE_L_Rear", "Wheel_42mm_ENVELOPE_L_Rear", "Axle_4mm_ENVELOPE_L_Rear", "BBB_22mm_Gearmotor_ENVELOPE_L_Front", "Wheel_42mm_ENVELOPE_L_Front", "Axle_4mm_ENVELOPE_L_Front", "BBB_22mm_Gearmotor_ENVELOPE_R_Rear", "Wheel_42mm_ENVELOPE_R_Rear", "Axle_4mm_ENVELOPE_R_Rear", "BBB_22mm_Gearmotor_ENVELOPE_R_Front", "Wheel_42mm_ENVELOPE_R_Front", "Axle_4mm_ENVELOPE_R_Front", "Replaceable_Side_Guard_L", "Replaceable_Side_Guard_R", "Plow_120mm_Replaceable", "Plow_Bolt_Land_L", "Plow_Bolt_Land_R", "Clamp_Jaw_Plate_6061", "Clamp_Downturned_Tip_6061", "Replaceable_Clamp_Tooth_1_Steel", "Replaceable_Clamp_Tooth_2_Steel", "Replaceable_Clamp_Tooth_3_Steel", "Clamp_Torque_Arm_L", "Clamp_Torque_Arm_R", "Hinge_Cheek_L", "Downward_Hard_Stop_L", "Hinge_Cheek_R", "Downward_Hard_Stop_R", "Hinge_Pin_6mm_ENVELOPE", "Repeat_40kg_Servo_ENVELOPE", "Servo_Output_Horn_6061", "Clamp_Linkage_L", "Clamp_Linkage_R", "Servo_Linkage_Sweep_ENVELOPE", "3S_Battery_104x35x27_ENVELOPE", "Dual_ESC_ENVELOPE", "Receiver_ENVELOPE", "UBEC_ENVELOPE", "Power_Switch_ENVELOPE", "Cover_Standoff_L_Rear", "Cover_Standoff_L_Front", "Cover_Standoff_R_Rear", "Cover_Standoff_R_Front", "Rear_Service_Lid_2mm", "Center_Service_Lid_2mm"
